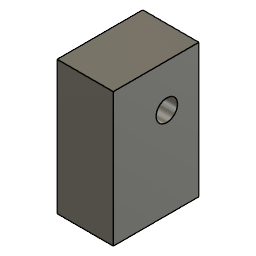
replay (Autodesk Fusion 360 design; units mm, degrees)
Autodesk Fusion 360 part; units mm, degrees
ref_plane "工作平面1" through (-15, 0, 0) normal (1, 0, 0) x (0, 1, 0)
sketch "草图1" plane through (-15, 0, 0) normal (1, 0, 0) x (0, 0, -1)
  line L0 (0, 50) -> (-32, 50)
  line L1 (-32, 50) -> (-32, 0)
  line L2 (-32, 0) -> (0, 0)
  line L3 (0, 0) -> (0, 50)
extrude "拉伸1" add sketch "草图1" along normal blind 21
sketch "草图2" plane through (6, 0, 0) normal (1, 0, 0) x (0, 0, -1)
  line L0 (0, 0) -> (0, 50)
  line L1 (0, 50) -> (-32, 50)
  line L2 (-32, 50) -> (-32, 0)
  line L3 (-32, 0) -> (0, 0)
  circle A0 centre (-12, 34) radius 4
extrude "拉伸2" cut sketch "草图2" against normal through all contours A0
